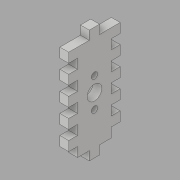
# Autodesk Inventor part: g_arm_v_2
Saved by Autodesk Inventor 2019 (Build 230136000, 136)
## iProperties
Created: 2021-11-02
Part Number: g_arm_v_2
Material: Generic
Document SubType Name: Modeling
Designer: Mohamed
Density: 1 g/cm^3
Appearance: Default
Author: Mohamed
Autodesk Inventor part; units mm, degrees
ref_plane "YZ Plane" through (0, 0, 0) normal (1, 0, 0) x (0, 1, 0)
ref_plane "XZ Plane" through (0, 0, 0) normal (0, 1, 0) x (-1, 0, 0)
ref_plane "XY Plane" through (0, 0, 0) normal (0, 0, 1) x (1, 0, 0)
sketch "Sketch1" plane through (0, 0, 0) normal (1, 0, 0) x (0, 1, 0)
  line L0 (0, 0) -> (65, 0)
  line L1 (65, -35) -> (0, -35)
  line L2 (65, -14) -> (71, -14)
  line L3 (71, -14) -> (71, -21)
  line L4 (71, -21) -> (65, -21)
  line L5 (0, -14) -> (-6, -14)
  line L6 (-6, -14) -> (-6, -21)
  line L7 (-6, -21) -> (0, -21)
  line L8 (65, 0) -> (65, -14)
  line L9 (65, -21) -> (65, -35)
  line L10 (0, -35) -> (0, -21)
  line L11 (0, -14) -> (0, 0)
  line L12 (32.5, -17.5) -> (22.5, -17.5)
  circle A0 centre (42.5, -17.5) radius 2.1
  circle A1 centre (22.5, -17.5) radius 2.1
  dimension "d0" = 65
  dimension "d1" = 35
  dimension "d3" = 6
  dimension "d4" = 7
  dimension "d6" = 6
  dimension "d7" = 7
  dimension "d8" = 10
  dimension "d10" = 4.2
  dimension "d11" = 4.2
  constraints: 26 end point, 8 perpendicular, 5 parallel, 2 centre point, 1 coincident, 1 horizontal
  measures "d0" distance of L1.start L1.end
  measures "d1" distance of L0.end L1.start
  measures "d3" distance of L2.start L2.end
  measures "d4" distance of L2.end L3.end
  measures "d6" distance of L5.start L5.end
  measures "d7" distance of L5.end L6.end
  measures "d8" distance of L12.start L12.end
  measures "d10" diameter of A0
  measures "d11" diameter of A1
extrude "Extrusion1" add sketch "Sketch1" along normal blind 6
sketch "Sketch2" plane through (6, 0, 0) normal (1, 0, 0) x (0, 0, -1)
  line L0 (14, 65) -> (0, 65) projected
  line L1 (0, 65) -> (0, 58.5)
  line L2 (0, 65) -> (0, 0) projected
  line L3 (0, 58.5) -> (6, 58.5)
  line L4 (6, 58.5) -> (6, 52)
  line L5 (6, 52) -> (0, 52)
  line L6 (0, 52) -> (0, 58.5)
  line L7 (35, 65) -> (35, 58.5)
  line L8 (35, 0) -> (35, 65) projected
  line L9 (35, 58.5) -> (29, 58.5)
  line L10 (29, 58.5) -> (29, 52)
  line L11 (29, 52) -> (35, 52)
  line L12 (35, 52) -> (35, 58.5)
  dimension "d15" = 6.5
  dimension "d16" = 6
  dimension "d17" = 6.5
  dimension "d18" = 6.5
  dimension "d19" = 6
  dimension "d20" = 6.5
  constraints: 20 end point, 4 parallel, 2 horizontal, 2 perpendicular, 2 point on line
  measures "d15" distance of L0.end L1.end
  measures "d16" distance of L4.end L5.end
  measures "d17" distance of L3.end L4.end
  measures "d18" distance of L7.start L7.end
  measures "d19" distance of L11.end L10.end
  measures "d20" distance of L10.end L9.end
extrude "Extrusion2" cut sketch "Sketch2" against normal blind 10
pattern_linear "Rectangular Pattern1" count 5 spacing 13 along (0, -1, 0) of "Extrusion2"
sketch "Sketch3" plane through (6, 0, 0) normal (1, 0, 0) x (0, 0, -1)
  circle A0 centre (17.5, 42.5) radius 2.1 projected
  circle A1 centre (17.5, 32.5) radius 5
  point P0 (0, 0)
  dimension "d27" = 10
  constraints: 1 centre point
  measures "d27" diameter of A1
extrude "Extrusion3" cut sketch "Sketch3" against normal blind 10 contours A1
body "Solid1"
